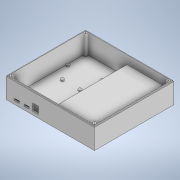
# Autodesk Inventor part: Couvercle inférieur
Saved by Autodesk Inventor 2020 (Build 240168000, 168)
## iProperties
Created: 2020-01-03
Part Number: Couvercle inférieur
Material: Générique
Document SubType Name: Modeling
Designer: Manuel Enzo
Density: 1 g/cm^3
Appearance: Par défaut
Author: Manuel Enzo
Autodesk Inventor part; units mm, degrees
ref_plane "YZ Plane" through (0, 0, 0) normal (1, 0, 0) x (0, 1, 0)
ref_plane "XZ Plane" through (0, 0, 0) normal (0, 1, 0) x (-1, 0, 0)
ref_plane "XY Plane" through (0, 0, 0) normal (0, 0, 1) x (1, 0, 0)
sketch "Esquisse1" plane through (0, 0, 0) normal (0, 1, 0) x (-1, 0, 0)
  line L0 (0, 0) -> (140, 0)
  line L1 (140, 0) -> (140, -126)
  line L2 (140, -126) -> (0, -126)
  line L3 (0, -126) -> (0, 0)
  line L4 (1, -1) -> (139, -1)
  line L5 (139, -1) -> (139, -125)
  line L6 (139, -125) -> (1, -125)
  line L7 (1, -125) -> (1, -1)
  line L8 (138, -2) -> (2, -2)
  line L9 (2, -2) -> (2, -124)
  line L10 (2, -124) -> (138, -124)
  line L11 (138, -124) -> (138, -2)
  circle A0 centre (135.5, -4.5) radius 2.5
  circle A1 centre (135.5, -4.5) radius 0.75
  circle A2 centre (135.5, -4.5) radius 1.5
  circle A3 centre (135.5, -121.5) radius 2.5
  circle A4 centre (135.5, -121.5) radius 1.5
  circle A5 centre (135.5, -121.5) radius 0.75
  circle A6 centre (4.5, -121.5) radius 2.5
  circle A7 centre (4.5, -121.5) radius 1.5
  circle A8 centre (4.5, -121.5) radius 0.75
  circle A9 centre (4.5, -4.5) radius 2.5
  circle A10 centre (4.5, -4.5) radius 1.5
  circle A11 centre (4.5, -4.5) radius 0.75
  circle A12 centre (135.25, -93.5) radius 2.5
  circle A13 centre (135.25, -93.5) radius 0.25
  circle A14 centre (87.25, -99.5) radius 2.5
  circle A15 centre (87.25, -99.5) radius 0.25
  circle A16 centre (135.25, -17.5) radius 2.5
  circle A17 centre (135.25, -17.5) radius 0.25
  circle A18 centre (87.25, -17.5) radius 2.5
  circle A19 centre (87.25, -17.5) radius 0.25
  circle A20 centre (119.75, -69) radius 2.5
  circle A21 centre (119.75, -69) radius 0.25
  circle A22 centre (91.75, -69) radius 2.5
  circle A23 centre (91.75, -69) radius 0.25
  line L12 (88.75, -14.5) -> (97.75, -14.5)
  line L13 (97.75, -14.5) -> (97.75, 0)
  line L14 (97.75, 0) -> (88.75, 0)
  line L15 (88.75, 0) -> (88.75, -14.5)
  line L16 (103.25, 0) -> (111.25, 0)
  line L17 (111.25, 0) -> (111.25, -6.5)
  line L18 (111.25, -6.5) -> (103.25, -6.5)
  line L19 (103.25, -6.5) -> (103.25, 0)
  line L20 (118.75, 0) -> (126.75, 0)
  line L21 (126.75, 0) -> (126.75, -6.5)
  line L22 (126.75, -6.5) -> (118.75, -6.5)
  line L23 (118.75, -6.5) -> (118.75, 0)
  line L24 (2, -2) -> (72, -2)
  line L25 (72, -2) -> (72, -124)
  line L26 (72, -124) -> (2, -124)
  line L27 (2, -124) -> (2, -2)
  point P0 (0, -11)
  point P1 (0, -19)
  point P2 (0, -26.5)
  point P3 (0, -34.5)
  point P4 (0, -40)
  point P5 (0, -49)
  point P6 (97.5, -53)
  point P7 (100, -50.5)
  point P8 (4.5, -2)
  point P9 (2, -4.5)
  point P10 (2, -121.5)
  point P11 (4.5, -124)
  point P12 (135.5, -124)
  point P13 (138, -121.5)
  point P14 (138, -4.5)
  point P15 (135.5, -2)
  point P16 (97.75, -2)
  point P17 (88.75, -2)
  point P18 (126.75, -2)
  point P19 (118.75, -2)
  point P20 (111.25, -2)
  point P21 (103.25, -2)
  dimension "d0" = 126
  dimension "d1" = 140
  dimension "d2" = 1
  dimension "d3" = 1
  dimension "d4" = 1
  dimension "d5" = 1
  dimension "d6" = 1
  dimension "d8" = 1
  dimension "d10" = 124
  dimension "d11" = 1
  dimension "d12" = 1
  dimension "d13" = 0.75
  dimension "d14" = 5
  dimension "d15" = 2.5
  dimension "d16" = 2.5
  dimension "d17" = 0.75
  dimension "d18" = 1
  dimension "d19" = 5
  dimension "d20" = 2.5
  dimension "d21" = 2.5
  dimension "d22" = 0.75
  dimension "d23" = 1
  dimension "d24" = 5
  dimension "d25" = 2.5
  dimension "d26" = 2.5
  dimension "d27" = 5
  dimension "d28" = 1
  dimension "d29" = 0.75
  dimension "d30" = 2.5
  dimension "d31" = 2.5
  dimension "d114" = 2.25
  dimension "d115" = 5
  dimension "d118" = 2.25
  dimension "d119" = 5
  dimension "d134" = 2.25
  dimension "d135" = 5
  dimension "d150" = 2.25
  dimension "d151" = 5
  dimension "d166" = 2.25
  dimension "d167" = 5
  dimension "d170" = 2.25
  dimension "d171" = 5
  dimension "d176" = 2.75
  dimension "d177" = 15.5
  dimension "d178" = 15.5
  dimension "d179" = 50.75
  dimension "d180" = 18.25
  dimension "d181" = 46.25
  dimension "d182" = 2.75
  dimension "d183" = 50.75
  dimension "d184" = 30.5
  dimension "d185" = 24.5
  dimension "d186" = 55
  dimension "d187" = 55
  dimension "d198" = 40.25
  dimension "d199" = 9
  dimension "d200" = 14.5
  dimension "d201" = 2
  dimension "d202" = 3
  dimension "d203" = 7.5
  dimension "d204" = 5.5
  dimension "d205" = 8
  dimension "d206" = 8
  dimension "d207" = 0
  constraints: 56 end point, 24 centre point, 14 coincident, 14 parallel, 7 horizontal, 7 perpendicular, 1 point on line
  measures "d0" distance between parallel lines of L0 L2
  measures "d1" distance between parallel lines of L3 L1
  measures "d2" distance between parallel lines of L5 L11
  measures "d3" distance between parallel lines of L10 L6
  measures "d4" distance between parallel lines of L7 L9
  measures "d5" distance between parallel lines of L8 L4
  measures "d6" distance between parallel lines of L3 L7
  measures "d8" distance between parallel lines of L6 L2
  measures "d10" distance of L6.end L4.start
  measures "d11" distance between parallel lines of L1 L5
  measures "d12" radial gap between concentric circles of A0 A2
  measures "d13" radial gap between concentric circles of A2 A1
  measures "d14" diameter of A0
  measures "d15" distance from line of L11 A0.centre
  measures "d16" distance from line of L8 A0.centre
  measures "d17" radial gap between concentric circles of A4 A5
  measures "d18" radial gap between concentric circles of A4 A3
  measures "d19" diameter of A3
  measures "d20" distance from line of A3.centre L11
  measures "d21" distance from line of A3.centre L10
  measures "d22" radial gap between concentric circles of A7 A8
  measures "d23" radial gap between concentric circles of A6 A7
  measures "d24" diameter of A6
  measures "d25" distance from line of A6.centre L10
  measures "d26" distance from line of A8.centre L9
  measures "d27" diameter of A9
  measures "d28" radial gap between concentric circles of A9 A10
  measures "d29" radial gap between concentric circles of A11 A10
  measures "d30" distance from line of L9 A10.centre
  measures "d31" distance from line of L8 A9.centre
  measures "d114" radial gap between concentric circles of A12 A13
  measures "d115" diameter of A12
  measures "d118" radial gap between concentric circles of A14 A15
  measures "d119" diameter of A14
  measures "d134" radial gap between concentric circles of A16 A17
  measures "d135" diameter of A16
  measures "d150" radial gap between concentric circles of A18 A19
  measures "d151" diameter of A18
  measures "d166" radial gap between concentric circles of A20 A21
  measures "d167" diameter of A20
  measures "d170" radial gap between concentric circles of A22 A23
  measures "d171" diameter of A22
  measures "d176" distance from line of L11 A16.centre
  measures "d177" distance from line of L8 A17.centre
  measures "d178" distance from line of L8 A18.centre
  measures "d179" distance from line of L11 A18.centre
  measures "d180" distance from line of L11 A20.centre
  measures "d181" distance from line of L11 A23.centre
  measures "d182" distance from line of L11 A13.centre
  measures "d183" distance from line of L11 A15.centre
  measures "d184" distance from line of L10 A13.centre
  measures "d185" distance from line of L10 A14.centre
  measures "d186" distance from line of L10 A22.centre
  measures "d187" distance from line of L10 A20.centre
  measures "d198" distance between parallel lines of L11 L13
  measures "d199" distance between parallel lines of L13 L15
  measures "d200" distance between parallel lines of L14 L12
  measures "d201" distance between parallel lines of L8 L14
  measures "d202" distance from line of A18.centre L12
  measures "d203" distance between parallel lines of L17 L23
  measures "d204" distance between parallel lines of L13 L19
  measures "d205" distance between parallel lines of L19 L17
  measures "d206" distance between parallel lines of L23 L21
  measures "d207" distance between parallel lines of L0 L16
extrude "Extrusion1" add sketch "Esquisse1" along normal blind 2 contours L15 L12 L13 L8 L19 L18 L17 L23 L22 L21 A0 L11 A3 L10 L25 | L8 L13 L12 L15 | L25 L10 A6 L9 A9 L8 | L8 L17 L18 L19 | A9 L9 L8 | L10 L9 A6 | A3 L11 L10 | L21 L22 L23 L8 | L8 L11 A0 | A13 | A15 | A17 | A19 | A21 | A23
extrude "Extrusion2" add sketch "Esquisse1" along normal blind 4 contours A12 | A14 | A16 | A18 | A20 | A22
extrude "Extrusion3" add sketch "Esquisse1" along normal blind 33.25 contours L15 L8 L9 L10 L11 L21 L4 L5 L6 L7 | L4 L13 L8 L15 | L4 L19 L8 L13 | L4 L17 L8 L19 | L4 L23 L8 L17 | A9 | L21 L8 L23 L4 | A6 | A3 | A0 | A2 | A4 | A7 | A10
extrude "Extrusion4" cut sketch "Esquisse1" along normal blind 32.25 contours A2 | A4 | A7 | A10
extrude "Extrusion5" add sketch "Esquisse1" along normal blind 31.75 contours L0 L15 L4 L7 L6 L5 L21 L1 L2 L3 | L0 L13 L4 L15 | L0 L19 L4 L13 | L0 L17 L4 L19 | L0 L23 L4 L17 | L21 L4 L23 L0
extrude "Extrusion6" add sketch "Esquisse1" along normal blind 16.5 contours L8 L13 L12 L15
extrude "Extrusion7" add sketch "Esquisse1" along normal blind 7 contours L8 L17 L18 L19 | L21 L22 L23 L8
sketch "Esquisse5" plane through (-88.75, 2, -14.5) normal (0, 0, -1) x (-1, 0, 0)
  line L0 (0, 0) -> (0, 14.5) projected
  line L1 (9, 0) -> (9, 14.5) projected
  line L2 (0, 14.5) -> (9, 14.5)
  line L3 (9, 14.5) -> (9, 3.5)
  line L4 (9, 3.5) -> (0, 3.5)
  line L5 (0, 3.5) -> (0, 14.5)
  line L6 (9, 0) -> (0, 0) projected
  line L7 (0, 3.5) -> (9, 3.5)
  line L8 (9, 3.5) -> (9, 0)
  line L9 (9, 0) -> (0, 0)
  line L10 (0, 0) -> (0, 3.5)
  point P0 (-88.75, -2)
  point P1 (0, 3.5)
  dimension "d215" = 11
  constraints: 16 end point, 4 parallel, 2 horizontal, 2 perpendicular, 1 point on line
  measures "d215" distance between parallel lines of L2 L4
extrude "Extrusion8" cut sketch "Esquisse5" against normal through all contours L0 L2 L1 L4
extrude "Extrusion9" cut sketch "Esquisse5" against normal blind 12.5 contours L0 L4 L1 L6
sketch "Esquisse6" plane through (-103.25, 2, -6.5) normal (0, 0, -1) x (-1, 0, 0)
  line L0 (8, 3.5) -> (0, 3.5)
  line L1 (23.5, 3.5) -> (15.5, 3.5)
  line L2 (0, 3.5) -> (8, 3.5)
  line L3 (8, 3.5) -> (8, 0)
  line L4 (0, 0) -> (0, 3.5)
  line L5 (23.5, 0) -> (15.5, 0) projected
  line L6 (15.5, 3.5) -> (23.5, 3.5)
  line L7 (23.5, 3.5) -> (23.5, 0)
  line L8 (23.5, 0) -> (15.5, 0)
  line L9 (15.5, 0) -> (15.5, 3.5)
  line L10 (8, 6.5) -> (0, 6.5)
  line L11 (23.5, 6.5) -> (15.5, 6.5)
  line L12 (8, 0) -> (0, 0) projected
  line L13 (0, 6.5) -> (0, 3.5)
  line L14 (0, 0) -> (0, 5) projected
  line L15 (8, 6.5) -> (8, 3.5)
  line L16 (8, 0) -> (8, 5) projected
  line L17 (15.5, 6.5) -> (15.5, 3.5)
  line L18 (23.5, 6.5) -> (23.5, 3.5)
  line L19 (23.5, 5) -> (23.5, 0) projected
  point P0 (-103.25, -2)
  point P1 (15.5, 5)
  dimension "d225" = 3.5
  dimension "d236" = 3.5
  dimension "d237" = 3
  dimension "d239" = 3
  dimension "d244" = 8
  dimension "d245" = 8
  dimension "d246" = 8
  dimension "d247" = 7.5
  constraints: 30 end point, 3 collinear, 3 parallel, 2 horizontal, 2 perpendicular, 1 point on line, 1 vertical
  measures "d225" distance between parallel lines of L1 L5
  measures "d236" distance between parallel lines of L12 L0
  measures "d237" distance between parallel lines of L0 L10
  measures "d239" distance between parallel lines of L11 L1
  measures "d244" distance between parallel lines of L3 L4
  measures "d245" distance between parallel lines of L9 L7
  measures "d246" distance between parallel lines of L17 L18
  measures "d247" distance between parallel lines of L3 L9
extrude "Extrusion12" cut sketch "Esquisse6" against normal through all contours L0 L13 L10 L15 | L1 L17 L11 L18
extrude "Extrusion13" cut sketch "Esquisse6" against normal blind 4.5 contours L3 L12 L4 L0 | L7 L5 L9 L1
extrude "Extrusion14" add sketch "Esquisse1" along normal blind 20 contours L25 L10 A6 L9 A9 L8 | A9 L9 L8 | L10 L9 A6
